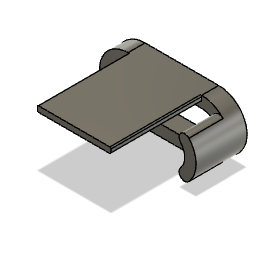
Hand_Left v4 (Autodesk Fusion 360 design; units mm, degrees)
Autodesk Fusion 360 part; units mm, degrees
note: some values were not read from the file. Set by a fixed rule: which sketch regions a step uses.
sketch "Sketch1" plane through (0, 0, 0) normal (0, 0, 1) x (1, 0, 0)
  line L0 (32.4286, -15) -> (-32.5714, -15)
  line L1 (-32.5714, 15) -> (32.4286, 15)
  arc A0 (-32.5714, 15) -> (-32.5714, -15) centre (-32.5714, 0) ccw
  arc A1 (32.4286, -15) -> (32.4286, 15) centre (32.4286, 0) ccw
  line L2 (-47.5714, 0) -> (47.4286, 0)
  line L3 (32.4286, -25) -> (-32.5714, -25)
  arc A2 (-32.5714, 25) -> (-32.5714, -25) centre (-32.5714, 0) ccw
  line L4 (-32.5714, 25) -> (32.4286, 25)
  arc A3 (32.4286, -25) -> (32.4286, 25) centre (32.4286, 0) ccw
  dimension "d7" = 30
  dimension "d8" = 65
  dimension "d9" = 10
  constraint horizontal L0
  constraint parallel L0 L1
  constraint midpoint A0 L2.start
  constraint midpoint A1 L2.end
  constraint horizontal L2
  constraint tangent L1 A0
  constraint tangent L1 A1
  constraint tangent L0 A0
  measures "d7" distance of L0.end L1.start
  measures "d8" distance of L1.start L1.end
extrude "Extrude1" add sketch "Sketch1" along normal blind 15
ref_plane "WorkPlane1" through (50, 0, 0) normal (1, 0, 0) x (0, 1, 0)
sketch "Sketch2" plane through (50, 0, 0) normal (1, 0, 0) x (0, 0, -1)
sketch "Sketch3" plane through (0, 0, 15) normal (0, 0, 1) x (1, 0, 0)
  arc A0 (-32.5714, 15) -> (-32.5714, -15) centre (-32.5714, 0) ccw
  line L0 (-32.5714, 15) -> (32.4286, 15)
  arc A1 (32.4286, -15) -> (32.4286, 15) centre (32.4286, 0) ccw
  line L1 (32.4286, -15) -> (-32.5714, -15)
  arc A2 (-32.5714, 25) -> (-32.5714, -25) centre (-32.5714, 0) ccw
  line L2 (-32.5714, -25) -> (32.4286, -25)
  arc A3 (32.4286, -25) -> (32.4286, 25) centre (32.4286, 0) ccw
  line L3 (32.4286, 25) -> (-32.5714, 25)
  arc A4 (51.1786, -16.5359) -> (51.1786, 16.5359) centre (32.4286, 0) ccw
  arc A5 (43.6786, -9.9216) -> (43.6786, 9.9216) centre (32.4286, 0) ccw
  arc A6 (48.5079, -18.1109) -> (51.1786, -16.5359) centre (47.4286, -13.2288) ccw
  arc A7 (43.6786, -9.9216) -> (48.5079, -18.1109) centre (47.4286, -13.2288) ccw
  arc A8 (51.1555, 16.5619) -> (43.6786, 9.9216) centre (47.4286, 13.2288) ccw
  arc A9 (51.1786, 16.5359) -> (51.1555, 16.5619) centre (47.4286, 13.2288) ccw
  dimension "d14" = 5
  dimension "d15" = 5
  dimension "d16" = 5
  dimension "d17" = 5
  dimension "d20" = 15
  dimension "d21" = 15
  constraint concentric A1 A4
  constraint concentric A1 A5
  constraint tangent A4 A6
  constraint tangent A5 A7
  constraint coincident A6.start A7.end
  constraint coincident L0.end A5
  constraint tangent A5 A8
  constraint tangent A4 A9
  constraint coincident A8.start A9.end
  constraint coincident A6.centre A7.centre
  constraint vertical A6.centre A8.centre
  measures "d14" radius of A6
  measures "d15" radius of A7
  measures "d16" radius of A8
  measures "d17" radius of A9
  measures "d20" horizontal distance of A3.end A8.centre
  measures "d21" horizontal distance of L2.end A6.centre
extrude "Extrude2" add sketch "Sketch3" along normal blind 30 contours A1 A3 A4 A5 A6 A7 A8 A9
sketch "Sketch4" plane through (0, 0, 15) normal (0, 0, 1) x (1, 0, 0)
  arc A0 (51.1786, 16.5359) -> (43.6786, 9.9216) centre (47.4286, 13.2288) ccw
  arc A1 (51.1786, 16.5359) -> (32.4286, 25) centre (32.4286, 0) ccw
  line L0 (32.4286, 25) -> (-32.5714, 25)
  arc A2 (-32.5714, 25) -> (-32.5714, -25) centre (-32.5714, 0) ccw
  line L1 (-32.5714, -25) -> (32.4286, -25)
  arc A3 (32.4286, -25) -> (51.1786, -16.5359) centre (32.4286, 0) ccw
  arc A4 (43.6786, -9.9216) -> (51.1786, -16.5359) centre (47.4286, -13.2288) ccw
  arc A5 (32.4286, -15) -> (43.6786, -9.9216) centre (32.4286, 0) ccw
  line L2 (32.4286, -15) -> (-32.5714, -15)
  arc A6 (-32.5714, 15) -> (-32.5714, -15) centre (-32.5714, 0) ccw
  line L3 (-32.5714, 15) -> (32.4286, 15)
  arc A7 (43.6786, 9.9216) -> (32.4286, 15) centre (32.4286, 0) ccw
  line L4 (-31.5714, 25) -> (31.4286, 25)
  line L5 (32.4286, 24) -> (32.4286, 21)
  line L6 (31.4286, 20) -> (-31.5714, 20)
  line L7 (-32.5714, 21) -> (-32.5714, 24)
  arc A8 (-32.5714, 21) -> (-31.5714, 20) centre (-31.5714, 21) ccw
  arc A9 (-31.5714, 25) -> (-32.5714, 24) centre (-31.5714, 24) ccw
  arc A10 (32.4286, 24) -> (31.4286, 25) centre (31.4286, 24) ccw
  arc A11 (31.4286, 20) -> (32.4286, 21) centre (31.4286, 21) ccw
  point P0 (-32.5714, 25)
  point P1 (-32.5714, 20)
  dimension "d22" = 5
  dimension "d25" = 1
  constraint horizontal L4
  constraint vertical L5
  constraint horizontal L6
  constraint vertical L7
  constraint coincident P0 L0.end
  constraint coincident P1 L6
  constraint coincident P1 L7
  constraint tangent L6 A8
  constraint tangent L7 A8
  constraint coincident P0 L4
  constraint coincident P0 L7
  constraint tangent L4 A9
  constraint tangent L7 A9
  constraint equal A8 A9
  constraint tangent L5 A10
  constraint tangent L4 A10
  constraint equal A8 A10
  constraint tangent L6 A11
  constraint tangent L5 A11
  constraint equal A8 A11
  measures "d22" distance of P0 P1
  measures "d25" radius of A8
extrude "Extrude3" add sketch "Sketch4" along normal blind 80 contours L0 L4 L5 L6 L7 A8 A9 A10 A11
ref_plane "WorkPlane2" through (50, 0, 0) normal (1, 0, 0) x (0, 1, 0)
sketch "Sketch5" plane through (50, 0, 0) normal (1, 0, 0) x (0, 0, -1)
  circle A0 centre (-37, 0) radius 5
extrude "Extrude4" [rolled back] along distance 12 taper angle 0
